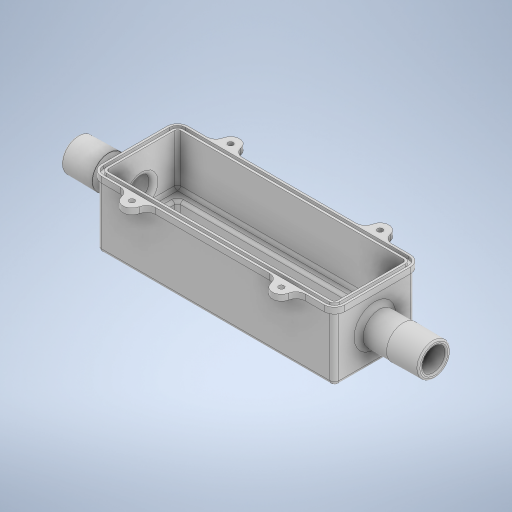
# Autodesk Inventor part: Rebreather-SensorEnclosure
Saved by Autodesk Inventor 2023 (Build 270158000, 158)
## iProperties
Created: 2022-11-09
Part Number: Rebreather-SensorEnclosure
Material: Generic
Document SubType Name: Modeling
Designer: incep
Density: 1 g/cm^3
Appearance: Default
Author: incep
## iProperties of the stored document Rebreather-SensorEnclosure_3DPrint.ipt
Created: 2022-11-09
Part Number: Rebreather-SensorEnclosure_3DPrint
Material: Generic
Document SubType Name: Modeling
Designer: incep
Density: 1 g/cm^3
Appearance: Default
Author: incep
Autodesk Inventor part; units mm, degrees
ref_plane "YZ Plane" through (0, 0, 0) normal (1, 0, 0) x (0, 1, 0)
ref_plane "XZ Plane" through (0, 0, 0) normal (0, 1, 0) x (-1, 0, 0)
sketch "Sketch1" plane through (0, 0, 0) normal (0, 1, 0) x (-1, 0, 0)
  line L0 (67.5, -15) -> (-67.5, -15) construction
  line L1 (-67.5, -15) -> (-67.5, 15) construction
  line L2 (-67.5, 15) -> (67.5, 15) construction
  line L3 (67.5, 15) -> (67.5, -15) construction
  line L4 (69.5, -17) -> (-69.5, -17)
  line L5 (-69.5, -17) -> (-69.5, 17)
  line L6 (-69.5, 17) -> (69.5, 17)
  line L7 (69.5, 17) -> (69.5, -17)
  line L8 (79.5, -27) -> (-79.5, -27)
  line L9 (-79.5, -27) -> (-79.5, 27)
  line L10 (-79.5, 27) -> (79.5, 27)
  line L11 (79.5, 27) -> (79.5, -27)
  line L12 (76.5, -24) -> (-76.5, -24)
  line L13 (-76.5, -24) -> (-76.5, 24)
  line L14 (-76.5, 24) -> (76.5, 24)
  line L15 (76.5, 24) -> (76.5, -24)
  point P0 (0, 0)
  point P1 (-67.5, 0)
  point P2 (0, -15)
  point P3 (-69.5, 0)
  point P4 (0, -17)
  point P5 (0, -27)
  point P6 (-79.5, 0)
  point P7 (0, -24)
  point P8 (-76.5, 0)
  dimension "d0" = 135
  dimension "d1" = 30
  dimension "d2" = 2
  dimension "d3" = 2
  dimension "d4" = 10
  dimension "d5" = 10
  dimension "d6" = 3
  dimension "d7" = 3
  constraints: 32 end point, 8 midpoint, 8 parallel, 4 horizontal, 4 horizontal alignment, 4 perpendicular, 4 vertical alignment
  measures "d0" distance of L1.end L2.end
  measures "d1" distance of L0.end L1.end
  measures "d2" distance between parallel lines of L7 L3
  measures "d3" distance between parallel lines of L4 L0
  measures "d4" distance between parallel lines of L11 L7
  measures "d5" distance between parallel lines of L8 L4
  measures "d6" distance between parallel lines of L15 L11
  measures "d7" distance between parallel lines of L8 L12
extrude "Extrusion1" add sketch "Sketch1" along normal blind 40 contours L8 L9 L10 L11
extrude "Extrusion2" add sketch "Sketch1" along normal blind 10 contours L12 L13 L14 L15
extrude "Extrusion3" add sketch "Sketch1" against normal blind 3 contours L4 L5 L6 L7 | L8 L9 L10 L11 | L12 L13 L14 L15
sketch "Sketch2" plane through (79.5, 40, 27) normal (1, 0, 0) x (0, 0, -1)
  line L0 (0, -43) -> (0, 0) projected
  line L1 (0, 0) -> (54, 0) projected
  line L2 (54, -43) -> (54, 0) projected
  line L3 (54, -40) -> (0, -40) projected
  line L4 (54, 0) -> (0, 0) construction
  line L5 (27, 0) -> (27, -40) construction
  line L6 (44, -40) -> (10, -40) construction
  line L7 (0, 0) -> (0, -43) construction
  line L8 (0, -20) -> (54, -20) construction
  line L9 (54, -43) -> (54, 0) construction
  point P0 (27, -20)
  point P1 (27, -20)
  constraints: 4 end point, 3 midpoint, 2 perpendicular, 2 point on line, 1 coincident
ref_plane "Work Plane1" through (-79.5, 40, 0) normal (0, 0, 1) x (1, 0, 0)
sketch "Sketch3" plane through (-79.5, 40, 0) normal (0, 0, 1) x (1, 0, 0)
  line L0 (199, -9.08) -> (159, -9.08) construction
  line L1 (159, -9.08) -> (159, -12.08)
  line L2 (159, -12.08) -> (199, -12.08)
  line L3 (199, -12.08) -> (199, -9.08)
  line L4 (159, -43) -> (159, 0) projected
  line L5 (199, -9.08) -> (178, -8.81)
  line L6 (178, -8.81) -> (178, -9.08)
  line L7 (178, -9.08) -> (159, -9.08)
  line L8 (159, -20) -> (238.0991, -20) construction
  point P0 (79.5, -40)
  dimension "d14" = 3
  dimension "d15" = 40
  dimension "d16" = 10.92
  dimension "d17" = 21
  dimension "d18" = 11.19
  constraints: 16 end point, 3 perpendicular, 2 horizontal, 2 parallel, 1 collinear, 1 point on line
  measures "d14" distance between parallel lines of L2 L0
  measures "d15" distance of L0.start L0.end
  measures "d16" vertical distance of L0.start L8.start
  measures "d17" horizontal distance of L5.end L0.start
  measures "d18" vertical distance of L8.start L5.end
revolve "Revolution1" add sketch "Sketch3" angle 360 about axis through (79.5, 20, 0) along (1, 0, 0)
sketch "Sketch4" plane through (79.5, 20, 0) normal (1, 0, 0) x (0, 0, -1)
  circle A0 centre (0, 0) radius 7.92 projected
  point P0 (0, -20)
extrude "Extrusion4" cut sketch "Sketch4" against normal up to surface (159 mm away)
mirror "Mirror1" about plane through (0, 0, 0) normal (1, 0, 0) of "Revolution1"
sketch "Sketch5" plane through (0, 40, 0) normal (0, 1, 0) x (1, 0, 0)
  line L0 (-81.5, 29) -> (81.5, 29)
  line L1 (81.5, 29) -> (81.5, -29)
  line L2 (81.5, -29) -> (-81.5, -29)
  line L3 (-81.5, -29) -> (-81.5, 29)
  line L4 (-76.5, 24) -> (76.5, 24) projected
  line L5 (-76.5, -24) -> (-76.5, 24) projected
  line L6 (76.5, -24) -> (-76.5, -24) projected
  line L7 (76.5, 24) -> (76.5, -24) projected
  point P0 (0, 0)
  point P1 (81.5, 0)
  point P2 (0, 29)
  dimension "d22" = 5
  dimension "d23" = 5
  constraints: 8 end point, 2 midpoint, 2 parallel, 1 horizontal, 1 horizontal alignment, 1 perpendicular, 1 vertical alignment
  measures "d22" distance between parallel lines of L0 L4
  measures "d23" distance between parallel lines of L3 L5
extrude "Extrusion5" add sketch "Sketch5" along normal blind 4
sketch "Sketch6" plane through (0, 44, 0) normal (0, 1, 0) x (1, 0, 0)
  line L0 (-81.5, 29) -> (-81.5, -29) projected
  line L1 (81.5, 29) -> (-81.5, 29) projected
  line L2 (81.5, -29) -> (81.5, 29) projected
  line L3 (-81.5, -29) -> (81.5, -29) projected
  line L4 (-80, 27.5) -> (80, 27.5)
  line L5 (80, 27.5) -> (80, -27.5)
  line L6 (80, -27.5) -> (-80, -27.5)
  line L7 (-80, -27.5) -> (-80, 27.5)
  line L8 (-78, 25.5) -> (78, 25.5)
  line L9 (78, 25.5) -> (78, -25.5)
  line L10 (78, -25.5) -> (-78, -25.5)
  line L11 (-78, -25.5) -> (-78, 25.5)
  point P0 (0, 0)
  point P1 (80, 0)
  point P2 (0, 27.5)
  point P3 (78, 0)
  point P4 (0, 25.5)
  dimension "d26" = 1.5
  dimension "d27" = 1.5
  dimension "d28" = 2
  dimension "d29" = 2
  constraints: 16 end point, 4 midpoint, 4 parallel, 2 horizontal, 2 horizontal alignment, 2 perpendicular, 2 vertical alignment
  measures "d26" distance between parallel lines of L0 L7
  measures "d27" distance between parallel lines of L1 L4
  measures "d28" distance between parallel lines of L4 L8
  measures "d29" distance between parallel lines of L7 L11
extrude "Extrusion6" cut sketch "Sketch6" against normal blind 2 contours L4 L5 L6 L7
sketch "Sketch7" plane through (0, 44, 0) normal (0, 1, 0) x (1, 0, 0)
  line L0 (-50, 33) -> (50, 33) construction
  line L1 (50, 33) -> (50, -33) construction
  line L2 (50, -33) -> (-50, -33) construction
  line L3 (-50, -33) -> (-50, 33) construction
  line L4 (-79.5, -27) -> (79.5, -27) construction
  circle A0 centre (-50, -33) radius 1.8
  circle A1 centre (-50, -33) radius 6 construction
  line L5 (-81.5, -29) -> (81.5, -29) projected
  line L6 (-54.4721, -29) -> (-45.5279, -29)
  arc A2 (-54.4721, -29) -> (-45.5279, -29) centre (-50, -33) ccw
  point P0 (0, 0)
  point P1 (50, 0)
  point P2 (0, 33)
  dimension "d32" = 100
  dimension "d33" = 6
  dimension "d34" = 3.6
  dimension "d37" = 33
  constraints: 10 end point, 4 point on circle, 3 centre point, 3 coincident, 2 midpoint, 2 parallel, 2 point on line, 1 concentric, 1 horizontal, 1 horizontal alignment, 1 perpendicular, 1 vertical alignment
  measures "d32" distance of L1.end L2.end
  measures "d33" distance between parallel lines of L2 L4
  measures "d34" diameter of A0
  measures "d37" vertical distance of L2.end point (0, 0)
extrude "Extrusion7" add sketch "Sketch7" against normal up to surface (4 mm away)
mirror "Mirror2" about plane through (0, 0, 0) normal (1, 0, 0) of "Extrusion7"
mirror "Mirror3" about plane through (0, 0, 0) normal (0, 0, 1) of "Extrusion7", "Mirror2"
fillet "Fillet1" radius 6 8 edges at (-54.4721, 42, -29) (-45.5279, 42, -29) (54.4721, 42, -29) (45.5279, 42, -29) (54.4721, 42, 29) (45.5279, 42, 29) (-45.5279, 42, 29) (-54.4721, 42, 29)
fillet "Fillet2" radius 3 10 edges at (-79.5, 18.5, 27) (-79.5, -3, 0) (-79.5, 18.5, -27) (0, -3, 27) (-79.5, 9.08, 0) (79.5, 18.5, 27) (79.5, -3, 0) (79.5, 18.5, -27) (79.5, 9.08, 0) (0, -3, -27)
fillet "Fillet3" radius 1 4 edges at (119.5, 9.08, 0) (-119.5, 9.08, 0) (-119.5, 12.08, 0) (119.5, 12.08, 0)
fillet "Fillet4" radius 2 16 edges at (76.5, 27, 24) (76.5, 27, -24) (-76.5, 27, 24) (-76.5, 27, -24) (0, 10, -24) (0, 10, 24) (-76.5, 10, 0) (76.5, 10, 0) (69.5, 5, -17) (69.5, 5, 17) (-69.5, 5, -17) (-69.5, 5, 17) (0, 10, -17) (69.5, 10, 0) (0, 10, 17) (-69.5, 10, 0)
fillet "Fillet5" radius 3.5 4 edges at (78, 43, 25.5) (78, 43, -25.5) (-78, 43, -25.5) (-78, 43, 25.5)
fillet "Fillet6" radius 5.5 4 edges at (80, 43, 27.5) (80, 43, -27.5) (-80, 43, 27.5) (-80, 43, -27.5)
fillet "Fillet7" radius 7 4 edges at (-81.5, 42, -29) (-81.5, 42, 29) (81.5, 42, -29) (81.5, 42, 29)
fillet "Fillet8" radius 3 2 edges at (76.5, 20, 7.92) (-76.5, 20, 7.92)
body "Solid1"
